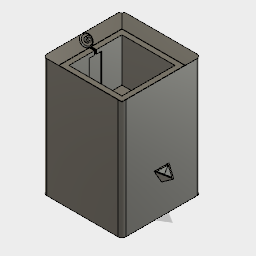
Pot-Desing v12 (Autodesk Fusion 360 design; units mm, degrees)
Autodesk Fusion 360 part; units mm, degrees
sketch "Sketch2" plane through (0, 0, 0) normal (0, 1, 0) x (1, 0, 0) in component "Outer-Box"
  line L0 (80, 80) -> (-80, 80)
  line L1 (-80, 80) -> (-80, -80)
  line L2 (-80, -80) -> (80, -80)
  line L3 (80, -80) -> (80, 80)
  line L4 (80, 80) -> (-80, -80) construction
  line L5 (-80, 80) -> (80, -80) construction
  dimension "d3" = 160
  dimension "d4" = 160
  measures "d3" distance of L1.end L2.end
  measures "d4" distance of L0.end L1.end
extrude "Extrude1" add sketch "Sketch2" along normal blind 240 makes body 1 in component "Outer-Box"
sketch "Sketch3" plane through (0, 240, 0) normal (0, 1, 0) x (-1, 0, 0) in component "Outer-Box"
  line L0 (-80, 80) -> (-80, -80)
  line L1 (-80, -80) -> (80, -80)
  line L2 (80, -80) -> (80, 80)
  line L3 (80, 80) -> (-80, 80)
  line L4 (64, 64) -> (-64, 64)
  line L5 (-64, 64) -> (-64, -64)
  line L6 (-64, -64) -> (64, -64)
  line L7 (64, -64) -> (64, 64)
  dimension "d7" = 16
extrude "Extrude2" cut sketch "Sketch3" against normal up to surface (224 mm away) contours L4 L5 L6 L7 bodies 1 in component "Outer-Box"
sketch "Sketch4" plane through (0, 240, 0) normal (0, 1, 0) x (-1, 0, 0) in component "Outer-Box"
  line L0 (64, -64) -> (-64, -64)
  line L1 (-64, -64) -> (-64, 64)
  line L2 (-64, 64) -> (64, 64)
  line L3 (64, 64) -> (64, -64)
  line L4 (-80, 80) -> (-80, -80)
  line L5 (-80, -80) -> (80, -80)
  line L6 (80, -80) -> (80, 80)
  line L7 (80, 80) -> (-80, 80)
  circle A0 centre (72, 0) radius 4
  point P0 (72, 0)
  dimension "d10" = 8
  measures "d10" diameter of A0
extrude "Extrude3" cut sketch "Sketch4" against normal up to surface (224 mm away) contours A0 bodies 1 in component "Outer-Box"
sketch "Sketch5" plane through (-64, 0, 0) normal (1, 0, 0) x (0, 0, -1) in component "Outer-Box"
  line L0 (-64, 16) -> (64, 16)
  line L1 (64, 16) -> (64, 240)
  line L2 (64, 240) -> (-64, 240)
  line L3 (-64, 240) -> (-64, 16)
  line L4 (4, 24) -> (-4, 24)
  line L5 (-4, 24) -> (-4, 16)
  line L6 (-4, 16) -> (4, 16)
  line L7 (4, 16) -> (4, 24)
  line L8 (4, 24) -> (-4, 16) construction
  line L9 (-4, 24) -> (4, 16) construction
  line L10 (4, 108.5) -> (-4, 108.5)
  line L11 (-4, 108.5) -> (-4, 93.5)
  line L12 (-4, 93.5) -> (4, 93.5)
  line L13 (4, 93.5) -> (4, 108.5)
  line L14 (4, 108.5) -> (-4, 93.5) construction
  line L15 (-4, 108.5) -> (4, 93.5) construction
  point P0 (0, 20)
  point P1 (0, 20)
  point P2 (0, 101)
  point P3 (0, 20)
  point P4 (0, 101)
  point P5 (0, 230)
  dimension "d14" = 8
  dimension "d15" = 8
  dimension "d16" = 15
  dimension "d17" = 8
  measures "d14" distance of L4.end L5.end
  measures "d15" distance of L5.end L6.end
  measures "d16" distance of L10.end L11.end
  measures "d17" distance of L11.end L12.end
extrude "Extrude4" cut sketch "Sketch5" against normal up to surface (8 mm away) contours L0 L4 L5 L6 L7 | L10 L11 L12 L13 bodies 1 in component "Outer-Box"
fillet "Fillet1" radius 4 6 edges at (-68, 108.5, -4) (-68, 108.5, 4) (-68, 93.5, 4) (-68, 93.5, -4) (-68, 24, 4) (-68, 24, -4) on bodies 1 in component "Outer-Box"
sketch "Sketch7" plane through (0, 16, 0) normal (0, 1, 0) x (-1, 0, 0) in component "Outer-Box"
  arc A0 (72, -4) -> (72, 4) centre (72, 0) ccw
  line L0 (72, 4) -> (64, 4)
  line L1 (64, 4) -> (64, 64)
  line L2 (64, 64) -> (-64, 64)
  line L3 (-64, 64) -> (-64, -64)
  line L4 (-64, -64) -> (64, -64)
  line L5 (64, -64) -> (64, -4)
  line L6 (64, -4) -> (72, -4)
  circle A1 centre (31, -31) radius 10
  circle A2 centre (-31, 30.9997) radius 10
  circle A3 centre (-31, -31) radius 10
  circle A4 centre (31, 30.9997) radius 10
  point P0 (31, -31)
  point P1 (-31, -31)
  point P2 (-31, -31)
  point P3 (-31, 30.9997)
  point P4 (31, 30.9997)
  dimension "d22" = 20
  dimension "d24" = 20
  dimension "d25" = 20
  dimension "d26" = 20
  measures "d22" diameter of A1
  measures "d24" diameter of A2
  measures "d25" diameter of A3
  measures "d26" diameter of A4
extrude "Extrude5" add sketch "Sketch7" along normal blind 50 contours A1 | A2 | A3 | A4 bodies 1 in component "Outer-Box"
chamfer "Chamfer2" distance 16 angle 45 4 edges at (-64, 240, 0) (0, 240, 64) (64, 240, 0) (0, 240, -64) on bodies 1 in component "Outer-Box"
fillet "Fillet2" radius 8 4 edges at (-80, 120, 80) (80, 120, 80) (80, 120, -80) (-80, 120, -80) on bodies 1 in component "Outer-Box"
ref_plane "WorkPlane1" through (0, 66, 0) normal (0, 1, 0) x (0, 0, 1) in component "Inner-Box-Electronics"
sketch "Sketch2 (2)" plane through (0, 66, 0) normal (0, 1, 0) x (1, 0, 0) in component "Inner-Box-Electronics"
  line L0 (63.5, 63.5) -> (-63.5, 63.5)
  line L1 (-63.5, 63.5) -> (-63.5, -63.5)
  line L2 (-63.5, -63.5) -> (63.5, -63.5)
  line L3 (63.5, -63.5) -> (63.5, 63.5)
  line L4 (63.5, 63.5) -> (-63.5, -63.5) construction
  line L5 (-63.5, 63.5) -> (63.5, -63.5) construction
  dimension "d32" = 127
  dimension "d33" = 127
  measures "d32" distance of L1.end L2.end
  measures "d33" distance of L0.end L1.end
extrude "Extrude1'" add sketch "Sketch2 (2)" along normal blind 60 separate body makes body 2 in component "Inner-Box-Electronics"
sketch "Sketch3 (2)" plane through (0, 126, 0) normal (0, 1, 0) x (-1, 0, 0) in component "Inner-Box-Electronics"
  line L0 (-63.5, 63.5) -> (-63.5, -63.5)
  line L1 (-63.5, -63.5) -> (63.5, -63.5)
  line L2 (63.5, -63.5) -> (63.5, 63.5)
  line L3 (63.5, 63.5) -> (-63.5, 63.5)
  line L4 (53.5, 53.5) -> (-53.5, 53.5)
  line L5 (-53.5, 53.5) -> (-53.5, -53.5)
  line L6 (-53.5, -53.5) -> (53.5, -53.5)
  line L7 (53.5, -53.5) -> (53.5, 53.5)
  dimension "d36" = 10
extrude "Extrude2'" cut sketch "Sketch3 (2)" against normal up to surface (50 mm away) contours L4 L5 L6 L7 bodies 2 in component "Inner-Box-Electronics"
sketch "Sketch4 (2)" plane through (-53.5, 0, 0) normal (1, 0, 0) x (0, 0, -1) in component "Inner-Box-Electronics"
  line L0 (-53.5, 76) -> (53.5, 76)
  line L1 (53.5, 76) -> (53.5, 126)
  line L2 (53.5, 126) -> (-53.5, 126)
  line L3 (-53.5, 126) -> (-53.5, 76)
  line L4 (4, 93.5) -> (-4, 93.5)
  line L5 (-4, 93.5) -> (-4, 108.5)
  line L6 (-4, 108.5) -> (4, 108.5)
  line L7 (4, 108.5) -> (4, 93.5)
  line L8 (4, 93.5) -> (-4, 108.5) construction
  line L9 (-4, 93.5) -> (4, 108.5) construction
  point P0 (0, 101)
  point P1 (0, 101)
  dimension "d39" = 15
  dimension "d40" = 8
  measures "d39" distance of L4.end L5.end
  measures "d40" distance of L5.end L6.end
extrude "Extrude3'" cut sketch "Sketch4 (2)" against normal blind 10 contours L4 L5 L6 L7 bodies 2 in component "Inner-Box-Electronics"
fillet "Fillet1'" radius 4 4 edges at (-58.5, 108.5, 4) (-58.5, 108.5, -4) (-58.5, 93.5, -4) (-58.5, 93.5, 4) on bodies 2 in component "Inner-Box-Electronics"
ref_plane "WorkPlane1" through (0, 126, 0) normal (0, 1, 0) x (0, 0, 1) in component "Inner-Box-Soil"
sketch "Sketch1" plane through (0, 126, 0) normal (0, 1, 0) x (1, 0, 0) in component "Inner-Box-Soil"
  line L0 (63.5, 63.5) -> (-63.5, 63.5)
  line L1 (-63.5, 63.5) -> (-63.5, -63.5)
  line L2 (-63.5, -63.5) -> (63.5, -63.5)
  line L3 (63.5, -63.5) -> (63.5, 63.5)
  line L4 (63.5, 63.5) -> (-63.5, -63.5) construction
  line L5 (-63.5, 63.5) -> (63.5, -63.5) construction
  dimension "d45" = 127
  dimension "d46" = 127
  measures "d45" distance of L1.end L2.end
  measures "d46" distance of L0.end L1.end
extrude "Extrude1''" add sketch "Sketch1" along normal blind 98 separate body makes body 3 in component "Inner-Box-Soil"
sketch "Sketch2 (3)" plane through (0, 224, 0) normal (0, 1, 0) x (-1, 0, 0) in component "Inner-Box-Soil"
  line L0 (-63.5, 63.5) -> (-63.5, -63.5)
  line L1 (-63.5, -63.5) -> (63.5, -63.5)
  line L2 (63.5, -63.5) -> (63.5, 63.5)
  line L3 (63.5, 63.5) -> (-63.5, 63.5)
  line L4 (53.5, 53.5) -> (-53.5, 53.5)
  line L5 (-53.5, 53.5) -> (-53.5, -53.5)
  line L6 (-53.5, -53.5) -> (53.5, -53.5)
  line L7 (53.5, -53.5) -> (53.5, 53.5)
  dimension "d49" = 10
extrude "Extrude2''" cut sketch "Sketch2 (3)" against normal up to surface (88 mm away) contours L4 L5 L6 L7 bodies 3 in component "Inner-Box-Soil"
sketch "Sketch6" plane through (-53.5, 0, 0) normal (1, 0, 0) x (0, 0, -1) in component "Inner-Box-Soil"
  line L0 (-53.5, 136) -> (53.5, 136)
  line L1 (53.5, 136) -> (53.5, 224)
  line L2 (53.5, 224) -> (-53.5, 224)
  line L3 (-53.5, 224) -> (-53.5, 136)
  line L4 (12.5, 216) -> (-12.5, 216)
  line L5 (-12.5, 216) -> (-12.5, 151)
  line L6 (-12.5, 151) -> (12.5, 151)
  line L7 (12.5, 151) -> (12.5, 216)
  line L8 (12.5, 216) -> (-12.5, 151) construction
  line L9 (-12.5, 216) -> (12.5, 151) construction
  line L10 (2, 224) -> (-2, 224)
  line L11 (-2, 224) -> (-2, 216)
  line L12 (-2, 216) -> (2, 216)
  line L13 (2, 216) -> (2, 224)
  line L14 (2, 224) -> (-2, 216) construction
  line L15 (-2, 224) -> (2, 216) construction
  point P0 (0, 183.5)
  point P1 (0, 183.5)
  point P2 (0, 220)
  point P3 (0, 220)
  dimension "d65" = 25
  dimension "d66" = 65
  dimension "d67" = 8
  dimension "d68" = 4
  measures "d65" distance of L5.end L6.end
  measures "d66" distance of L4.end L5.end
  measures "d67" distance of L10.end L11.end
  measures "d68" distance of L11.end L12.end
extrude "Extrude7" cut sketch "Sketch6" against normal blind 2 contours L2 L4 L10 L11 L12 L13 | L4 L5 L6 L7 L12 bodies 3 in component "Inner-Box-Soil"
sketch "Sketch7 (2)" plane through (0, 224, 0) normal (0, 1, 0) x (-1, 0, 0) in component "Inner-Box-Soil"
  line L0 (55.5, -2) -> (53.5, -2)
  line L1 (53.5, -2) -> (53.5, -53.5)
  line L2 (53.5, -53.5) -> (-53.5, -53.5)
  line L3 (-53.5, -53.5) -> (-53.5, 53.5)
  line L4 (-53.5, 53.5) -> (53.5, 53.5)
  line L5 (53.5, 53.5) -> (53.5, 2)
  line L6 (53.5, 2) -> (55.5, 2)
  line L7 (55.5, 2) -> (55.5, -2)
  line L8 (-63.5, 63.5) -> (-63.5, -63.5)
  line L9 (-63.5, -63.5) -> (63.5, -63.5)
  line L10 (63.5, -63.5) -> (63.5, 63.5)
  line L11 (63.5, 63.5) -> (-63.5, 63.5)
  line L12 (55.5, -2) -> (63.5, -2)
  line L13 (63.5, -2) -> (63.5, 2)
  line L14 (63.5, 2) -> (55.5, 2)
  line L15 (55.5, 2) -> (55.5, -2)
  line L16 (55.5, -2) -> (63.5, 2) construction
  line L17 (63.5, -2) -> (55.5, 2) construction
  point P0 (59.5, 0)
  point P1 (59.5, 0)
extrude "Extrude8" cut sketch "Sketch7 (2)" against normal blind 2 contours L7 L10 L12 L13 L14 L15 bodies 3 in component "Inner-Box-Soil"
sketch "Sketch11" plane through (80, 80, 0) normal (0.707107, 0.707107, 0) x (0, 0, -1) in component "Outer-Box"
  ellipse E0 centre (0, 214.9605) end of major axis (0, 220.6173) minor radius 4
  ellipse E1 centre (72, 214.9605) end of major axis (72, 226.2742) minor radius 8 (77.6569, 222.9605) -> (72, 226.2742) ccw
  line L0 (72, 226.2742) -> (-72, 226.2742)
  ellipse E2 centre (-72, 214.9605) end of major axis (-72, 226.2742) minor radius 8 (-72, 226.2742) -> (-77.6569, 222.9605) ccw
  line L1 (-77.6569, 222.9605) -> (-64, 203.6468)
  line L2 (-64, 203.6468) -> (64, 203.6468)
  line L3 (64, 203.6468) -> (77.6569, 222.9605)
  line L4 (-1.9926, 203.6468) -> (2.0074, 203.6468)
  line L5 (2.0074, 203.6468) -> (2.0074, 210.0462)
  line L6 (2.0074, 210.0462) -> (-1.9926, 210.0462)
  line L7 (-1.9926, 210.0462) -> (-1.9926, 203.6468)
extrude "Extrude6" cut sketch "Sketch11" against normal blind 2 contours E0 L2 L4 L5 L6 L7 bodies 1 in component "Outer-Box"
chamfer "Chamfer3" distance 2 angle 45 1 edges at (-64, 224, -0.0074) on bodies 1 in component "Outer-Box"
sketch "Sketch13" plane through (80, 0, 0) normal (1, 0, 0) x (0, 0, -1) in component "Outer-Box"
  line L0 (72, 0) -> (72, 240)
  line L1 (72, 240) -> (-72, 240)
  line L2 (-72, 240) -> (-72, 0)
  line L3 (-72, 0) -> (72, 0)
  line L4 (-14.9996, 86) -> (0, 60.02)
  line L5 (0, 60.02) -> (14.9996, 86)
  line L6 (14.9996, 86) -> (-14.9996, 86)
  point P0 (0, 77.34)
  point P1 (0, 77.34)
extrude "Extrude8'" add sketch "Sketch13" along normal blind 30 draft -19.47 contours L4 L5 L6 bodies 1 in component "Outer-Box"
sketch "Sketch14" plane through (35.9136, 101.5858, 0) normal (0.333313, 0.942816, 0) x (0, 0, -1) in component "Outer-Box"
  line L0 (-14.9996, -46.7604) -> (0, -72.7419)
  line L1 (0, -72.7419) -> (14.9996, -46.7604)
  line L2 (14.9996, -46.7604) -> (-14.9996, -46.7604)
  line L3 (0, -68.7417) -> (11.5356, -48.7604)
  line L4 (11.5356, -48.7604) -> (-11.5356, -48.7604)
  line L5 (-11.5356, -48.7604) -> (0, -68.7417)
  dimension "d82" = 2
extrude "Extrude9" cut sketch "Sketch14" against normal blind 33 draft -19.47 contours L3 L4 L5 bodies 1 in component "Outer-Box"
sketch "Sketch15" plane through (81.8856, 0, 0) normal (1, 0, 0) x (0, 0, -1) in component "Outer-Box"
  line L0 (0, 65.3514) -> (11.5356, 85.3334)
  line L1 (11.5356, 85.3334) -> (-11.5356, 85.3334)
  line L2 (-11.5356, 85.3334) -> (0, 65.3514)
  line L3 (-11.5356, 85.3334) -> (0, 65.3532)
  line L4 (0, 65.3532) -> (11.5356, 85.3334)
  line L5 (11.5356, 85.3334) -> (-11.5356, 85.3334)
  point P0 (0, 78.6733)
extrude "Extrude10" cut sketch "Sketch15" against normal up to surface (17.8856 mm away) draft 3.5 bodies 1 in component "Outer-Box"
ref_plane "WorkPlane1" through (-72, 232, 0) normal (0.707107, 0.707107, 0) x (0, 0, -1) in component "Sprout"
sketch "Sketch1 (2)" plane through (-72, 232, 0) normal (0.707107, 0.707107, 0) x (0, 0, -1) in component "Sprout"
  circle A0 centre (0, 0) radius 11.3137
  line L0 (72, 11.3137) -> (-72, 11.3137)
extrude "Extrude1'''" add sketch "Sketch1 (2)" along normal blind 2 draft -45 separate body makes body 4 in component "Sprout"
sketch "Sketch3 (3)" plane through (81.4142, 81.4142, 0) normal (0.707107, 0.707107, 0) x (0, 0, -1) in component "Sprout"
  circle A0 centre (0, 214.9605) radius 9.3137
  circle A1 centre (0, 214.9605) radius 4.9997
  dimension "d94" = 4.314
extrude "Extrude3''" add sketch "Sketch3 (3)" along normal blind 6 contours A1 bodies 4 in component "Sprout"
sketch "Sketch4 (3)" plane through (85.6569, 85.6569, 0) normal (0.707107, 0.707107, 0) x (0, 0, -1) in component "Sprout"
  circle A0 centre (0, 214.9605) radius 4.9997
  circle A1 centre (0, 214.9605) radius 2.7497
  dimension "d97" = 2.25
extrude "Extrude4'" cut sketch "Sketch4 (3)" against normal up to surface (8 mm away) contours A1 bodies 4 in component "Sprout"
sketch "Sketch16" plane through (0, 0, -64) normal (0, 0, 1) x (1, 0, 0) in component "Outer-Box"
  line L0 (64, 224) -> (-64, 224)
  line L1 (-64, 224) -> (-64, 16)
  line L2 (-64, 16) -> (64, 16)
  line L3 (64, 16) -> (64, 224)
  circle A0 centre (0, 110) radius 6
  point P0 (0, 110)
  dimension "d100" = 12
  measures "d100" diameter of A0
extrude "Extrude11" cut sketch "Sketch16" against normal up to surface (16 mm away) contours A0 bodies 1 in component "Outer-Box"
sketch "Sketch5 (2)" plane through (0, 0, -53.5) normal (0, 0, 1) x (1, 0, 0) in component "Inner-Box-Electronics"
  line L0 (-53.5, 76) -> (53.5, 76)
  line L1 (53.5, 76) -> (53.5, 126)
  line L2 (53.5, 126) -> (-53.5, 126)
  line L3 (-53.5, 126) -> (-53.5, 76)
  circle A0 centre (0, 110) radius 6
  point P0 (0, 110)
  dimension "d103" = 12
  measures "d103" diameter of A0
extrude "Extrude4''" cut sketch "Sketch5 (2)" against normal up to surface (10 mm away) contours A0 bodies 2 in component "Inner-Box-Electronics"
component "Outer-Box" placed x (1, 0, 0) y (0, 1, 0) z (0, 0, 1) at (0, 0, 0)
component "Inner-Box-Electronics" placed x (1, 0, 0) y (0, 1, 0) z (0, 0, 1) at (0, 0, 0)
component "Inner-Box-Soil" placed x (1, 0, 0) y (0, 1, 0) z (0, 0, 1) at (0, 0, 0)
component "Sprout" placed x (1, 0, 0) y (0, 1, 0) z (0, 0, 1) at (0, 0, 0)
component "View" placed x (1, 0, 0) y (0, 1, 0) z (0, 0, 1) at (0, 0, 0)
